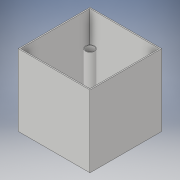
# Autodesk Inventor part: sebis-1
Saved by Autodesk Inventor 2019.1 (Build 231200000, 200)
## iProperties
Created: 2018-12-18
Part Number: sebis-1
Material: 一般
Document SubType Name: Modeling
Designer: Masaya
Density: 1 g/cm^3
Appearance: 既定
Author: Masaya
Autodesk Inventor part; units mm, degrees
ref_plane "YZ Plane" through (0, 0, 0) normal (1, 0, 0) x (0, 1, 0)
ref_plane "XZ Plane" through (0, 0, 0) normal (0, 1, 0) x (-1, 0, 0)
ref_plane "XY Plane" through (0, 0, 0) normal (0, 0, 1) x (1, 0, 0)
sketch "スケッチ1" plane through (0, 0, 0) normal (0, 1, 0) x (-1, 0, 0)
  line L0 (0, 0) -> (310, 0)
  line L1 (310, 0) -> (310, 310)
  line L2 (310, 310) -> (0, 310)
  line L3 (0, 310) -> (0, 0)
  dimension "d0" = 310
  dimension "d1" = 310
  constraints: 8 end point, 2 parallel, 1 horizontal, 1 perpendicular
  measures "d0" distance of L1.end L2.end
  measures "d1" distance of L0.end L1.end
extrude "押し出し1" add sketch "スケッチ1" along normal blind 10
sketch "スケッチ2" plane through (0, 10, 0) normal (0, 1, 0) x (1, 0, 0)
  line L0 (-305, -305) -> (-5, -305)
  line L1 (-5, -305) -> (-5, -5)
  line L2 (-5, -5) -> (-305, -5)
  line L3 (-305, -5) -> (-305, -305)
  line L4 (-310, 0) -> (-310, -310) projected
  line L5 (-310, -310) -> (0, -310) projected
  line L6 (0, 0) -> (-310, 0) projected
  line L7 (-310, 0) -> (-310, -310) projected
  line L8 (-310, -310) -> (0, -310) projected
  line L9 (0, -310) -> (0, 0) projected
  dimension "d4" = 300
  dimension "d5" = 300
  dimension "d6" = 5
  dimension "d7" = 5
  constraints: 8 end point, 2 parallel, 1 horizontal, 1 perpendicular
  measures "d4" distance of L2.end L1.end
  measures "d5" distance of L1.end L0.end
  measures "d6" distance between parallel lines of L3 L4
  measures "d7" distance between parallel lines of L0 L5
extrude "押し出し2" add sketch "スケッチ2" along normal blind 300
sketch "スケッチ3" plane through (0, 10, 0) normal (0, 1, 0) x (1, 0, 0)
  circle A0 centre (-155, -155) radius 20
  line L0 (-305, -305) -> (-305, -5) projected
  line L1 (-5, -305) -> (-305, -305) projected
  circle A1 centre (-155, -155) radius 17.5
  point P0 (0, 0)
  dimension "d10" = 40
  dimension "d11" = 150
  dimension "d12" = 150
  dimension "d13" = 35
  constraints: 2 centre point, 1 coincident
  measures "d10" diameter of A0
  measures "d11" distance from line of L0 A0.centre
  measures "d12" distance from line of L1 A0.centre
  measures "d13" diameter of A1
extrude "押し出し3" add sketch "スケッチ3" along normal blind 300
